Autodesk Fusion 360 part; units mm, degrees
(part 2 of 2)
sketch "Sketch7 (3)" plane through (0, 0, 3) normal (0, 0, 1) x (-1, 0, 0) in component "ServoHolder"
  line L0 (-102.9854, 154.0365) -> (-102.9854, 113.0365)
  line L1 (-102.9854, 113.0365) -> (-61.9854, 113.0365)
  line L2 (-61.9854, 113.0365) -> (-61.9854, 154.0365)
  line L3 (-61.9854, 154.0365) -> (-102.9854, 154.0365)
  circle A0 centre (-68.9854, 144.0365) radius 1
  circle A1 centre (-82.4854, 133.5365) radius 4
  circle A2 centre (-68.9854, 123.0365) radius 1
  circle A3 centre (-95.9854, 144.0365) radius 1
  circle A4 centre (-95.9854, 123.0365) radius 1
  line L4 (-82.4854, 133.5365) -> (-78.4854, 133.5365) construction
  line L5 (-82.4854, 133.5365) -> (-76.4575, 127.5086) construction
  circle A5 centre (-77.5356, 128.5868) radius 1.5
  circle A6 centre (-77.5356, 138.4863) radius 1.5
  circle A7 centre (-87.4351, 138.4863) radius 1.5
  circle A8 centre (-87.4351, 128.5868) radius 1.5
  dimension "d246" = 135
  dimension "d247" = 3
  dimension "d248" = 7
  dimension "d250" = 360
  constraint coincident A1.centre L4.start
  constraint coincident A1 L4.end
  constraint horizontal L4
  constraint coincident L5 A5.centre
  measures "d246" angle of L4 L5
  measures "d247" diameter of A5
  measures "d248" distance of A1.centre A5.centre
extrude "Extrude7''" cut sketch "Sketch7 (3)" against normal blind 3 contours A5 | A6 | A7 | A8 bodies 3 in component "ServoHolder"
sketch "Sketch2 (6)" plane through (0, 0, 3) normal (0, 0, 1) x (-1, 0, 0) in component "Base Plate"
  circle A0 centre (-196.915, -54) radius 1.5
  circle A1 centre (-196.915, 54) radius 1.5
  circle A2 centre (0, -50.9117) radius 2
  circle A3 centre (-50.9117, 0) radius 2
  circle A4 centre (0, 50.9117) radius 2
  circle A5 centre (50.9117, 0) radius 2
  circle A6 centre (-50.9117, 50.9117) radius 1.5
  circle A7 centre (-50.9117, -50.9117) radius 1.5
  circle A8 centre (0, 72) radius 1.5
  circle A9 centre (72, 0) radius 1.5
  circle A10 centre (50.9117, -50.9117) radius 1.5
  circle A11 centre (0, -72) radius 1.5
  circle A12 centre (50.9117, 50.9117) radius 1.5
  arc A13 (-199.915, 60) -> (-202.915, 57) centre (-199.915, 57) ccw
  line L0 (-202.915, 57) -> (-202.915, -57)
  arc A14 (-202.915, -57) -> (-199.915, -60) centre (-199.915, -57) ccw
  line L1 (-199.915, -60) -> (-52.915, -60)
  arc A15 (-52.915, -60) -> (-52.915, 60) centre (0, 0) ccw
  line L2 (-52.915, 60) -> (-199.915, 60)
sketch "Sketch8 (2)" plane through (0, 0, 3) normal (0, 0, 1) x (-1, 0, 0) in component "SquareUConnector"
  circle A0 centre (54.5117, 132.4157) radius 4
  line L0 (67.0117, 151.9157) -> (42.0117, 151.9157)
  line L1 (42.0117, 151.9157) -> (42.0117, 112.9157)
  line L2 (42.0117, 112.9157) -> (67.0117, 112.9157)
  line L3 (67.0117, 112.9157) -> (67.0117, 151.9157)
  line L4 (54.5117, 132.4157) -> (46.6071, 132.4157) construction
  line L5 (54.5117, 132.4157) -> (48.1965, 126.1005) construction
  circle A1 centre (49.562, 127.466) radius 1.5
  circle A2 centre (59.4615, 127.466) radius 1.5
  circle A3 centre (59.4615, 137.3655) radius 1.5
  circle A4 centre (49.562, 137.3655) radius 1.5
  dimension "d253" = 45
  dimension "d254" = 3
  dimension "d255" = 7
  dimension "d257" = 360
  constraint coincident A0.centre L4.start
  constraint horizontal L4
  constraint coincident L5 A1.centre
  measures "d253" angle of L4 L5
  measures "d254" diameter of A1
  measures "d255" distance of A0.centre A1.centre
extrude "Extrude9" cut sketch "Sketch8 (2)" against normal blind 3 contours A1 | A2 | A3 | A4 bodies 7 in component "SquareUConnector"
sketch "Sketch4 (6)" plane through (0, 0, 3) normal (0, 0, 1) x (-1, 0, 0) in component "ServoCutOut"
  line L0 (12.8865, 167.6678) -> (12.8865, 158.6678)
  arc A0 (12.8865, 155.6678) -> (12.8865, 158.6678) centre (12.8865, 157.1678) ccw
  line L1 (12.8865, 155.6678) -> (12.8865, 146.6678)
  line L2 (12.8865, 146.6678) -> (-28.1135, 146.6678)
  line L3 (-28.1135, 146.6678) -> (-28.1135, 155.6678)
  arc A1 (-28.1135, 158.6678) -> (-28.1135, 155.6678) centre (-28.1135, 157.1678) ccw
  line L4 (-28.1135, 158.6678) -> (-28.1135, 167.6678)
  line L5 (-28.1135, 167.6678) -> (12.8865, 167.6678)
  circle A2 centre (16.8865, 161.1678) radius 2
  circle A3 centre (-32.1135, 153.1678) radius 2
  circle A4 centre (16.8865, 153.1678) radius 2
  circle A5 centre (-32.1135, 161.1678) radius 2
  circle A6 centre (2.8865, 157.1678) radius 60
  circle A7 centre (2.8865, 157.1678) radius 72 construction
  line L6 (2.8865, 157.1678) -> (-69.1135, 157.1678) construction
  line L7 (2.8865, 157.1678) -> (-48.0252, 106.2561) construction
  line L8 (-48.0252, 106.2561) -> (-48.0252, 157.1678) construction
  circle A8 centre (-48.0252, 157.1678) radius 2
  circle A9 centre (2.8865, 106.2561) radius 2
  circle A10 centre (53.7982, 157.1678) radius 2
  circle A11 centre (2.8865, 208.0795) radius 2
  dimension "d260" = 144
  dimension "d261" = 45
  dimension "d262" = 4
  dimension "d264" = 360
  constraint concentric A6 A7
  constraint coincident A6.centre A7.centre
  constraint coincident A7 L6.end
  constraint horizontal L6
  constraint coincident A7 L7.end
  constraint coincident L6 L8.end
  constraint perpendicular L6 L8
  constraint coincident L8.end A8.centre
  measures "d260" diameter of A7
  measures "d261" angle of L6 L7
  measures "d262" diameter of A8
extrude "Extrude5'''" cut sketch "Sketch4 (6)" against normal blind 3 contours A8 | A9 | A10 | A11 bodies 4 in component "ServoCutOut"
sketch "Sketch2 (7)" plane through (0, 0, 6) normal (0, 0, 1) x (-1, 0, 0) in component "BearingOutside"
  circle A0 centre (2.8865, 157.1678) radius 45
  circle A1 centre (2.8865, 157.1678) radius 60
  circle A2 centre (2.8865, 157.1678) radius 72 construction
  line L0 (2.8865, 157.1678) -> (-69.1135, 157.1678) construction
  line L1 (2.8865, 157.1678) -> (-48.0252, 106.2561) construction
  line L2 (-48.0252, 106.2561) -> (-48.0252, 157.1678) construction
  circle A3 centre (-48.0252, 157.1678) radius 2
  circle A4 centre (2.8865, 106.2561) radius 2
  circle A5 centre (53.7982, 157.1678) radius 2
  circle A6 centre (2.8865, 208.0795) radius 2
  dimension "d267" = 144
  dimension "d268" = 45
  dimension "d269" = 4
  dimension "d271" = 360
  constraint concentric A0 A2
  constraint coincident A0.centre A1.centre
  constraint coincident A2 L0.end
  constraint horizontal L0
  constraint coincident A2 L1.end
  constraint coincident L0 L2.end
  constraint perpendicular L0 L2
  constraint coincident L2.end A3.centre
  measures "d267" diameter of A2
  measures "d268" angle of L0 L1
  measures "d269" diameter of A3
extrude "Extrude2''''''" cut sketch "Sketch2 (7)" against normal blind 3 contours A3 | A4 | A5 | A6 bodies 5 in component "BearingOutside"
sketch "dxf" plane through (-94.9754, -122.7327, 41) normal (0, 1, 0) x (-1, 0, 0) in component "CustomConnection"
  circle A0 centre (-11.1758, -20.5) radius 1
  circle A1 centre (-3.1758, -16.5) radius 1
  circle A2 centre (-10.2485, -10.7652) radius 1
  line L0 (-17.2826, -25.0836) -> (-11.8943, -8.5)
  circle A3 centre (3.8969, -10.7652) radius 1
  circle A4 centre (4.8242, -20.5) radius 1
  line L1 (-3.1758, -35.3328) -> (-17.2826, -25.0836)
  circle A5 centre (-3.1758, -24.5) radius 1
  line L2 (5.5427, -8.5) -> (10.931, -25.0836)
  circle A6 centre (-3.1758, -32.5328) radius 1
  line L3 (10.931, -25.0836) -> (-3.1758, -35.3328)
  line L4 (-11.8943, -8.5) -> (5.5427, -8.5)
  circle A7 centre (-14.6197, -24.2183) radius 1
  circle A8 centre (8.2681, -24.2183) radius 1
  line L5 (-24.1758, -41) -> (17.8242, -41)
  line L6 (17.8242, -41) -> (17.8242, -30)
  line L7 (17.8242, -30) -> (25.8242, -30)
  line L8 (25.8242, -30) -> (25.8242, -6)
  line L9 (25.8242, -6) -> (17.3242, -6)
  line L10 (17.3242, -6) -> (17.3242, 0)
  line L11 (17.3242, 0) -> (-23.6758, 0)
  line L12 (-23.6758, 0) -> (-23.6758, -6)
  line L13 (-23.6758, -6) -> (-32.1758, -6)
  line L14 (-32.1758, -6) -> (-32.1758, -30)
  line L15 (-32.1758, -30) -> (-24.1758, -30)
  line L16 (-24.1758, -30) -> (-24.1758, -41)
  line L17 (-11.8943, -8.5) -> (3.8776, -30.2082) construction
  line L18 (5.5427, -8.5) -> (-10.2292, -30.2082) construction
  line L19 (-3.1758, -41) -> (-3.1758, 0) construction
  line L20 (-3.1758, -20.5) -> (-32.1758, -20.5) construction
  line L21 (-3.1758, -20.5) -> (25.8242, -20.5) construction
  point P0 (-3.1758, -20.5)
  constraint midpoint L3 L17.end
  constraint perpendicular L3 L17
  constraint midpoint L1 L18.end
  constraint perpendicular L1 L18
  constraint coincident L17 P0
  constraint coincident L18 P0
  constraint midpoint L5 L19.start
  constraint midpoint L11 L19.end
  constraint midpoint L19 P0
  constraint coincident L14 L20.end
  constraint perpendicular L14 L20
  constraint coincident L8 L21.end
  constraint perpendicular L8 L21
  constraint coincident P0 L20.start
extrude "Extrude9'" cut sketch "dxf" against normal blind 3 contours A0 | A1 | A4 | A5 bodies 8 in component "CustomConnection"
component "Base Plate" placed x (1, 0, 0) y (0, 1, 0) z (0, 0, 1) at (-52.915, 60, 0)
component "CircularL" placed x (1, 0, 0) y (0, 1, 0) z (0, 0, 1) at (83.3982, 250.8664, 0)
component "ServoHolder" placed x (0, -1, 0) y (1, 0, 0) z (0, 0, 1) at (265.0365, 43.9854, 0)
component "ServoCutOut" placed x (1, 0, 0) y (0, 1, 0) z (0, 0, 1) at (222.8865, 121.6678, 0)
component "BearingOutside" placed x (1, 0, 0) y (0, 1, 0) z (0, 0, 1) at (217.8865, -17.8322, -3)
component "UConnector" placed x (1, 0, 0) y (0, 1, 0) z (0, 0, 1) at (126.0772, 32.7415, 0)
component "SquareUConnector" placed x (1, 0, 0) y (0, 1, 0) z (0, 0, 1) at (143.0117, 79.9157, 0)
component "CustomConnection" placed x (1, 0, 0) y (0, 0, 1) z (0, -1, 0) at (174.7996, -85, 149.7327)
component "Pentagon Connection" placed x (1, 0, 0) y (0, 1, 0) z (0, 0, 1) at (91.9493, 68.4454, 0)
equation "Thick = 3 mm"
equation "d6 = h3"
equation "h3 = 3 mm"
equation "d8 = 6.5 mm + h3 / 2"
equation "d13 = h4"
equation "d18 = Thick"
equation "d20 = h3"
equation "d21 = h3 * 2"
equation "d22 = h3 * 2"
equation "d23 = h3"
equation "d24 = h3 * 2"
equation "d25 = h3 * 2"
equation "d26 = Thick"
equation "h2 = 2 mm"
equation "h4 = 4 mm"
equation "d32 = h4"
equation "d33 = 0.5 mm + h4"
equation "d36 = h4"
equation "d37 = h4 * 3"
equation "d38 = h4"
equation "d39 = 3 * h4"
equation "d41 = h3"
equation "d42 = 4 mm + h3"
equation "d46 = 12.5 mm + h2 / 2"
equation "d49 = Thick"
equation "d54 = h2"
equation "d55 = 10 mm + h2 / 2"
equation "d56 = 7 mm + h2 / 2"
equation "d57 = Thick"
equation "d61 = Thick"
equation "d65 = 13 mm - Thick"
equation "d73 = h2"
equation "d74 = h2"
equation "d75 = h2"
equation "d76 = 2 mm + h2"
equation "d77 = 1.5 mm + h2 / 2"
equation "d78 = 1.5 mm + h2 / 2"
equation "d79 = 13 mm + h2"
equation "ServoL = 41 mm"
equation "ServoW = 21 mm"
equation "widthToCenter = 10 mm"
equation "d100 = -Thick"
equation "d102 = h2"
equation "d103 = h2"
equation "d104 = h2"
equation "d105 = h2"
equation "d106 = -Thick"
equation "d109 = Thick"
equation "d115 = -Thick"
equation "d117 = ServoL"
equation "d118 = ServoW"
equation "d119 = widthToCenter"
equation "d122 = -Thick"
equation "d124 = h4"
equation "d125 = h4 / 2 + 2 mm"
equation "d126 = h4 / 2 + 2 mm"
equation "d127 = -Thick"
equation "d129 = 120 mm - 30 mm"
equation "d130 = Thick"
equation "d134 = Thick"
equation "d136 = Thick"
equation "d137 = Thick"
equation "d141 = ( 25 / 2 ) * 1 mm"
equation "d143 = h3"
equation "d144 = 4 mm + 1.5 mm + h3 / 2"
equation "d150 = h3"
equation "d151 = 5.5 mm + h3 / 2"
equation "d155 = h2"
equation "d156 = 4 mm + 2 mm + h2 / 2"
equation "d159 = -Thick"
equation "d163 = 42 mm + Thick"
equation "d164 = 24 mm + Thick"
equation "d165 = Thick"
equation "d169 = Thick"
equation "d171 = Thick"
equation "d172 = Thick"
equation "d173 = 26 mm - Thick"
equation "d176 = ( 25 / 2 ) * 1 mm"
equation "d178 = h2"
equation "d179 = 6 mm + h2 / 2"
equation "d186 = h2"
equation "d187 = 3 mm + h2 / 2"
equation "d188 = 1 mm + h2 / 2"
equation "d189 = h2"
equation "d190 = -Thick"
equation "d194 = -Thick"
equation "d200 = -Thick"
equation "d202 = 24 mm + Thick"
equation "d204 = Thick"
equation "d206 = Thick"
equation "d210 = Thick"
equation "d214 = Thick"
equation "d221 = h4"
equation "d222 = h4"
equation "d223 = 4.5 mm + h4 / 2"
equation "d224 = h4 + 6.2 mm"
equation "d225 = -Thick"
equation "d227 = h3"
equation "d228 = 10.5 mm + h3 / 2"
equation "d229 = 9.2 mm + h3 / 2"
equation "d230 = -Thick"
equation "d233 = Thick"
equation "d239 = -Thick"
equation "d242 = h2"
equation "d243 = 9 mm + h3 / 2"
equation "d244 = -Thick"
equation "d247 = h3"
equation "d248 = 5.5 mm + h3 / 2"
equation "d251 = -Thick"
equation "d254 = h3"
equation "d255 = 5.5 mm + h3 / 2"
equation "d258 = -Thick"
equation "d262 = h4"
equation "d265 = -Thick"
equation "d269 = h4"
equation "d272 = -Thick"
equation "d274 = -Thick"
